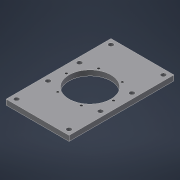
# Autodesk Inventor part: P017-Carter_chapeau
Saved by Autodesk Inventor 2021.3 (Build 253353000, 353)
## iProperties
Created: 2022-04-01
Part Number: P017-Carter_chapeau
Material: Générique
Document SubType Name: Modeling
Designer: remi
Density: 1 g/cm^3
Appearance: Par défaut
Author: remi
Autodesk Inventor part; units mm, degrees
ref_plane "YZ Plane" through (0, 0, 0) normal (1, 0, 0) x (0, 1, 0)
ref_plane "XZ Plane" through (0, 0, 0) normal (0, 1, 0) x (-1, 0, 0)
ref_plane "XY Plane" through (0, 0, 0) normal (0, 0, 1) x (1, 0, 0)
sketch "Sketch2" plane through (0, 0, 0) normal (0, 0, 1) x (1, 0, 0)
  line L0 (-30, -50) -> (30, -50)
  line L1 (30, -50) -> (30, 50)
  line L2 (30, 50) -> (-30, 50)
  line L3 (-30, 50) -> (-30, -50)
  line L4 (-30, -50) -> (30, 50) construction
  line L5 (30, -50) -> (-30, 50) construction
  point P0 (0, 0)
  dimension "d0" = 60
  dimension "d1" = 100
  constraints: 12 end point, 2 midpoint, 2 parallel, 1 horizontal, 1 perpendicular
  measures "d0" distance of L1.end L2.end
  measures "d1" distance of L0.end L1.end
extrude "Extrusion1" add sketch "Sketch2" along normal blind 5
sketch "Sketch3" plane through (0, 0, 5) normal (0, 0, 1) x (1, 0, 0)
  circle A0 centre (0, 0) radius 20
  line L0 (-30, 50) -> (-30, -50) construction
  line L1 (30, -50) -> (30, 50) construction
  line L2 (30, 50) -> (-30, 50) construction
  line L3 (-30, 50) -> (-30, -50) construction
  line L4 (-30, -50) -> (30, -50) construction
  dimension "d5" = 60
  dimension "d6" = 40
  constraints: 1 centre point, 1 coincident
  measures "d5" distance of L1.end L2.end
  measures "d6" diameter of A0
extrude "Extrusion2" cut sketch "Sketch3" against normal blind 5
sketch "Sketch6" plane through (0, 0, 5) normal (0, 0, 1) x (1, 0, 0)
  line L0 (30, -50) -> (30, 50) construction
  line L1 (30, 50) -> (-30, 50) construction
  line L2 (-30, 50) -> (-30, -50) construction
  line L3 (-30, -50) -> (30, -50) construction
  line L4 (20, -40) -> (-20, -40) construction
  line L5 (-20, -40) -> (-20, 40) construction
  line L6 (-20, 40) -> (20, 40) construction
  line L7 (20, 40) -> (20, -40) construction
  circle A0 centre (25, -15) radius 1.621 projected
  circle A1 centre (-25, 15) radius 1.621 projected
  circle A2 centre (-25, 45) radius 1.621 projected
  circle A3 centre (25, -45) radius 1.621 projected
  circle A4 centre (-25, -45) radius 1.621 projected
  circle A5 centre (25, 45) radius 1.621 projected
  circle A6 centre (-25, -15) radius 1.621 projected
  circle A7 centre (25, 15) radius 1.621 projected
  point P0 (0, 0)
  point P1 (-25, -45)
  point P2 (-25, -15)
  point P3 (-25, 15)
  point P4 (-25, 45)
  point P5 (25, 45)
  point P6 (25, 15)
  point P7 (25, -15)
  point P8 (25, -45)
hole "Hole3" at (-25, -45, 5) at (-25, -15, 5) at (-25, 15, 5) at (-25, 45, 5) at (25, 45, 5) at (25, 15, 5) at (25, -15, 5) at (25, -45, 5) direction (0, 0, -1) diameter 4.5 end through all clearance for "Flat Head Machine Screw" size "M4" standard "Ansi Metric M Profile"
sketch "Sketch7" plane through (0, 0, 5) normal (0, 0, 1) x (1, 0, 0)
  circle A0 centre (0, 0) radius 25 construction
  circle A1 centre (0, 0) radius 20 construction
  line L0 (-42, 0) -> (42, 0) construction
  circle A2 centre (0, 0) radius 22.5 construction
  point P0 (-22.5, 0)
  point P1 (-11.25, -19.4856)
  point P2 (11.25, -19.4856)
  point P3 (22.5, 0)
  point P4 (11.25, 19.4856)
  point P5 (-11.25, 19.4856)
  dimension "d43" = 45
  dimension "d41" = 50
  dimension "d42" = 40
  dimension "d46" = 360
  constraints: 1 coincident, 1 horizontal alignment, 1 point on line, 9 other
  measures "d41" diameter of A0
  measures "d42" diameter of A1
hole "Hole4" at (-22.5, 0, 5) at (-11.25, -19.4856, 5) at (11.25, -19.4856, 5) at (22.5, 0, 5) at (11.25, 19.4856, 5) at (-11.25, 19.4856, 5) direction (0, 0, -1) diameter 2.459 end through all thread size "M3x0.5" class "6H" standard "ISO Metric profile"
equation "\"d43\" = 0.5 * d41 + 0.5 * d42"
body "Solid1"
